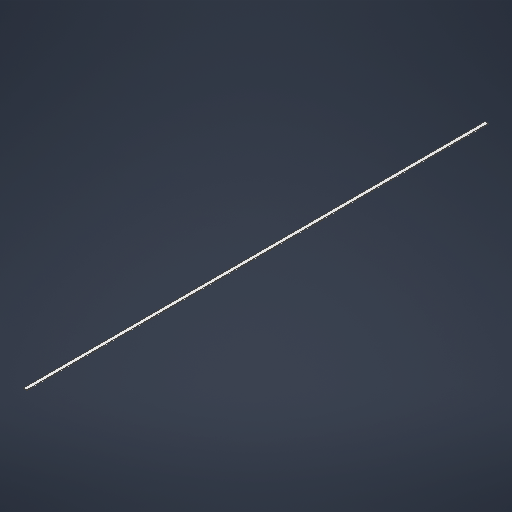
# Autodesk Inventor part: SP40-13 REVESTIMIENTO - LAMA FIJA TUBULAR
Saved by Autodesk Inventor 2025 (Build 290162000, 162)
## iProperties
Created: 2026-01-30
Part Number: SP40-13 REVESTIMIENTO - LAMA FIJA TUBULAR
Material: Aluminio
Document SubType Name: Modeling
Designer: ROLANDO
Density: 2.7 g/cm^3
Appearance: Satinado
Author: ROLANDO
Autodesk Inventor part; units mm, degrees
ref_plane "YZ Plane" through (0, 0, 0) normal (1, 0, 0) x (0, 1, 0)
ref_plane "XZ Plane" through (0, 0, 0) normal (0, 1, 0) x (-1, 0, 0)
ref_plane "XY Plane" through (0, 0, 0) normal (0, 0, 1) x (1, 0, 0)
sketch "Boceto1" plane through (0, 0, 0) normal (0, 0, 1) x (1, 0, 0)
  line L0 (0, 0) -> (37, 0)
  line L1 (37, 8) -> (0, 8)
  line L2 (0, 1.3) -> (37, 1.3)
  line L3 (37, 6.7) -> (0, 6.7)
  arc A0 (0, 6.7) -> (0, 1.3) centre (0, 4) ccw
  line L4 (-8.2346, 4) -> (45.2882, 4) construction
  arc A1 (0, 8) -> (0, 0) centre (0, 4) ccw
  arc A2 (37, 0) -> (37, 8) centre (37, 4) ccw
  arc A3 (37, 1.3) -> (37, 6.7) centre (37, 4) ccw
  point P0 (41, 4)
  point P1 (-4, 4)
  dimension "d1" = 1.3
  dimension "d2" = 1.3
  dimension "d5" = 8
  dimension "d10" = 4
  dimension "d11" = 1.3
  dimension "d12" = 4
  dimension "d13" = 2.7
  dimension "d16" = 1.3
  dimension "d17" = 2.7
  dimension "d18" = 4
  dimension "d19" = 45
  constraints: 10 end point, 10 point on circle, 4 centre point, 3 coincident, 3 horizontal, 2 parallel, 2 point on line
  measures "d1" distance between parallel lines of L2 L0
  measures "d2" distance between parallel lines of L1 L3
  measures "d5" distance between parallel lines of L1 L0
  measures "d10" distance between parallel lines of L1 L4
  measures "d11" radial gap between concentric circles of A1 A0
  measures "d12" radius of A1
  measures "d13" radius of A0
  measures "d16" radial gap between concentric circles of A2 A3
  measures "d17" radius of A3
  measures "d18" radius of A2
  measures "d19" distance of point (41, 4) point (-4, 4)
extrude "Extrusión1" add sketch "Boceto1" against normal blind 5000
